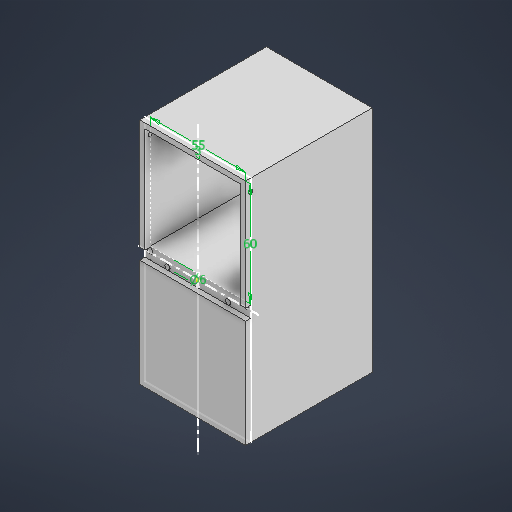
# Autodesk Inventor part: frame
Saved by Autodesk Inventor 2025.3 (Build 293356030, 356C)
## iProperties
Created: 2025-12-14
Part Number: frame
Material: 一般
Document SubType Name: Modeling
Designer: 陳泓任
Density: 1 g/cm^3
Appearance: 預設
Author: 陳泓任
Autodesk Inventor part; units mm, degrees
ref_plane "YZ Plane" through (0, 0, 0) normal (1, 0, 0) x (0, 1, 0)
ref_plane "XZ Plane" through (0, 0, 0) normal (0, 1, 0) x (-1, 0, 0)
ref_plane "XY Plane" through (0, 0, 0) normal (0, 0, 1) x (1, 0, 0)
sketch "草圖1" plane through (0, 0, 0) normal (0, 0, 1) x (1, 0, 0)
  line L0 (-27.5, 3) -> (27.5, 3) construction
  line L1 (27.5, 3) -> (27.5, 63) construction
  line L2 (27.5, 63) -> (-27.5, 63) construction
  line L3 (-27.5, 63) -> (-27.5, 3) construction
  line L4 (-30.5, 66) -> (30.5, 66)
  line L5 (30.5, 66) -> (30.5, -5.5597)
  line L6 (-30.5, -3) -> (-30.5, 66)
  line L7 (-34.7579, 0) -> (34.7579, 0)
  line L8 (-30.5, -66) -> (30.5, -66)
  line L9 (30.5, -66) -> (30.5, -5.5597)
  line L10 (-30.5, -3) -> (-30.5, -66)
  line L11 (0, 77.5612) -> (0, -87.4517)
  point P0 (0, 3)
  point P1 (0, 3)
  point P2 (0, -3)
  point P3 (0, 0)
  dimension "d0" = 55
  dimension "d1" = 60
  dimension "d2" = 3
  dimension "d3" = 6
  constraints: 24 end point, 3 parallel, 3 symmetric about line, 2 midpoint, 1 coincident, 1 horizontal, 1 perpendicular, 1 point on line, 1 vertical, 3 other
  measures "d0" distance of L2.end L1.end
  measures "d1" distance of L1.end L0.end
  measures "d2" distance between parallel lines of L2 L4
  measures "d3" diameter of L0 L7
extrude "擠出1" add sketch "草圖1" along normal blind 3 and the other way blind 70
shell "薄殼1" thickness 3 removed faces 1 at (-10.1667, 22, -70)
sketch "草圖2" plane through (0, 0, 0) normal (0, 0, 1) x (1, 0, 0)
  line L0 (27.5, 63) -> (27.5, -4)
  line L1 (27.5, -4) -> (-27.5, -4)
  line L2 (-27.5, -4) -> (-27.5, 63)
  line L3 (0, 77.5612) -> (0, -87.4517) projected
  line L4 (-34.7579, 0) -> (34.7579, 0) projected
  line L5 (27.5, 63) -> (-27.5, 63) projected
  point P0 (0, 0)
  point P1 (-27.5, 0)
  point P2 (27.5, 0)
  dimension "d8" = 55
  dimension "d9" = 8
  constraints: 6 end point, 2 point on line, 1 parallel, 1 other
  measures "d8" distance between parallel lines of L0 L2
  measures "d9" diameter of L1 L4
extrude "擠出2" cut sketch "草圖2" along normal blind 3 and the other way blind 2
sketch "草圖3" plane through (0, 0, 0) normal (1, 0, 0) x (0, 1, 0)
  circle A0 centre (59, 0) radius 1.25
  line L0 (-66, 3) -> (66, 3) projected
  line L1 (-4, 0) -> (-4, 3) construction
  line L2 (2, 0) -> (2, 3) construction
  dimension "d13" = 2.5
  dimension "d17" = 3
  dimension "d20" = 6
  dimension "d21" = 57
  constraints: 2 end point, 1 centre point, 1 point on line, 1 vertical
  measures "d13" diameter of A0
  measures "d17" distance from line of A0.centre L0
  measures "d20" distance between parallel lines of L1 L2
  measures "d21" distance from line of A0.centre L2
extrude "擠出3" cut sketch "草圖3" along normal through all both and the other way through all
sketch "草圖4" plane through (0, 0, 0) normal (1, 0, 0) x (0, 1, 0)
  line L0 (66, -70) -> (-66, -70) projected
  line L1 (1.4687, -70) -> (0, -70)
  line L2 (77.5612, 0) -> (-87.4517, 0) projected
  line L3 (3, 1) -> (3, -70)
  line L4 (3, -70) -> (-1, -70)
  line L5 (-1, -70) -> (-1, 1)
  line L6 (-4, 0) -> (-4, 3) projected
  line L7 (3, 1) -> (-1, 1)
  point P0 (0, 0)
  point P1 (3, 0)
  point P2 (3, 0)
  point P3 (3, 0)
  dimension "d39" = 71
  dimension "d40" = 4
  constraints: 11 end point, 2 horizontal, 2 point on line, 2 vertical, 1 collinear
  measures "d39" distance between parallel lines of L0 L7
  measures "d40" distance of L3.start L5.end
extrude "擠出4" add sketch "草圖4" along normal mid plane 55
sketch "草圖5" plane through (0, 0, 3) normal (0, 0, 1) x (1, 0, 0)
  line L0 (-30.5, 66) -> (-30.5, -66) projected
  line L1 (-30.5, -4) -> (30.5, -4)
  line L2 (30.5, -4) -> (30.5, 2.5)
  line L3 (-30.5, 2.5) -> (-30.5, -4)
  line L4 (27.5, -4) -> (-27.5, -4) projected
  line L5 (30.5, -66) -> (30.5, 66) projected
  circle A0 centre (-27.5, 0.7) radius 1.25 construction
  line L6 (-27.5, 3) -> (27.5, 3) projected
  line L7 (-27.5, 3) -> (27.5, 3)
  line L8 (27.5, 3) -> (27.5, 2.5)
  line L9 (-27.5, 2.5) -> (-27.5, 3)
  line L10 (-30.5, 2.5) -> (-27.5, 2.5)
  line L11 (27.5, 2.5) -> (30.5, 2.5)
  line L12 (27.5, 63) -> (27.5, -4) construction
  point P0 (0, 0)
  dimension "d41" = 2.5
  dimension "d42" = 3
  dimension "d46" = 6.5
  constraints: 16 end point, 4 collinear, 4 horizontal, 3 perpendicular, 2 parallel, 1 centre point, 1 point on line
  measures "d41" diameter of A0
  measures "d42" distance from line of L0 A0.centre
  measures "d46" distance between parallel lines of L1 L10
extrude "擠出5" cut sketch "草圖5" against normal blind 3
sketch "草圖6" plane through (-27.5, -63, 0) normal (1, 0, 0) x (0, 0, -1)
  line L0 (0, 63) -> (3, 63)
  line L1 (3, 63) -> (3, 59)
  line L2 (3, 59) -> (0, 59)
  line L3 (0, 59) -> (0, 63)
  line L4 (-3, 59) -> (0, 59) projected
  dimension "d37" = 3
  constraints: 8 end point, 2 parallel, 1 collinear, 1 horizontal, 1 perpendicular
  measures "d37" distance of L0.start L0.end
extrude "擠出6" add sketch "草圖6" along normal up to surface (55 mm away)
sketch "草圖7" plane through (-30.5, -4, 0) normal (0, 0, 1) x (1, 0, 0)
  circle A0 centre (3, 4.7) radius 1.5
  circle A1 centre (13, 1.5) radius 1.5
  line L0 (61, 0) -> (0, 0) projected
  line L1 (30.5, 81.5612) -> (30.5, -83.4517) projected
  circle A2 centre (58, 4.7) radius 1.5
  circle A3 centre (48, 1.5) radius 1.5
  line L2 (0, 0) -> (0, 6.5) projected
  line L3 (0, 6.5) -> (3, 6.5) projected
  point P0 (30.5, 4)
  point P1 (0, 4)
  point P2 (58, 0)
  dimension "d30" = 3
  dimension "d31" = 3
  dimension "d32" = 35
  dimension "d38" = 3
  dimension "d45" = 1.8
  constraints: 4 centre point, 2 symmetric about line, 1 tangent, 2 other
  measures "d30" diameter of A1
  measures "d31" diameter of A0
  measures "d32" diameter of A1.centre L1
  measures "d38" distance from line of L2 A0.centre
  measures "d45" distance from line of A0.centre L3
extrude "擠出7" cut sketch "草圖7" against normal blind 3
equation "\"d8\" = d0"
